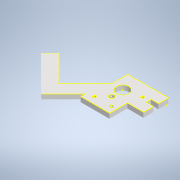
# Autodesk Inventor part: gripper laser cut
Saved by Autodesk Inventor 2020.1 (Build 241239000, 239)
## iProperties
Created: 2019-10-24
Part Number: gripper laser cut
Material: Generic
Document SubType Name: Modeling
Designer: amirs
Density: 1 g/cm^3
Appearance: Default
Author: amirs
Autodesk Inventor part; units mm, degrees
ref_plane "YZ Plane" through (0, 0, 0) normal (1, 0, 0) x (0, 1, 0)
ref_plane "XZ Plane" through (0, 0, 0) normal (0, 1, 0) x (-1, 0, 0)
ref_plane "XY Plane" through (0, 0, 0) normal (0, 0, 1) x (1, 0, 0)
sketch "Sketch1" plane through (0, 0, 0) normal (0, 1, 0) x (-1, 0, 0)
  line L0 (51.5704, 31.4309) -> (74.021, 53.8815)
  line L1 (74.021, 53.8815) -> (109.942, 17.9605)
  line L2 (109.942, 17.9605) -> (100.9618, 8.9803)
  line L3 (100.9618, 8.9803) -> (74.021, 35.921)
  line L4 (74.021, 35.921) -> (47.0803, 8.9803)
  line L5 (100.9618, 8.9803) -> (107.5624, 2.3796) construction
  line L6 (35.9043, 29.2241) -> (44.6165, 29.2241) construction
  line L7 (35.9043, 29.2241) -> (27.1921, 29.2241) construction
  circle A0 centre (44.6165, 29.2241) radius 1.5263
  circle A1 centre (27.1921, 29.2241) radius 1.6891
  circle A2 centre (35.9043, 20.4103) radius 2.54
  circle A3 centre (35.9043, 8.9803) radius 6.35
  line L8 (51.5704, 31.4309) -> (51.5704, 36.1902)
  line L9 (51.5704, 36.1902) -> (22.0986, 36.1902)
  line L10 (22.0986, 36.1902) -> (22.0986, 17.9605)
  line L11 (47.0803, 8.9803) -> (47.0803, 0)
  line L12 (5.5886, 17.9605) -> (22.0986, 17.9605)
  line L13 (5.5886, 17.9605) -> (5.5886, -7.4395)
  line L14 (5.5886, -7.4395) -> (47.0803, -7.4395)
  line L15 (47.0803, -7.4395) -> (47.0803, 0)
  point P0 (0, 0)
  dimension "d1" = 12.7
  dimension "d3" = 38.1
  dimension "d5" = 12.7
  dimension "d19" = 8.7122
  dimension "d20" = 8.7122
  dimension "d23" = 5.08
  dimension "d24" = 25.4
  dimension "d38" = 16.51
  dimension "d39" = 29.4718
  constraints: 32 end point, 7 perpendicular, 4 centre point, 3 vertical, 2 coincident, 2 horizontal, 1 parallel, 1 point on line
  measures "d1" distance between parallel lines of L4 L0
  measures "d3" distance of L2.end L3.end
  measures "d5" distance between parallel lines of L1 L3
  measures "d19" distance of L6.start L6.end
  measures "d20" distance of L6.start L7.end
  measures "d23" diameter of A2
  measures "d24" distance of L12.start L13.end
  measures "d38" distance of L12.start L10.end
  measures "d39" distance between parallel lines of L8 L10
extrude "Extrusion1" add sketch "Sketch1" along normal blind 5.08
sketch "Sketch2" plane through (0, 5.08, 0) normal (0, 1, 0) x (1, 0, 0)
  line L0 (-5.5886, -17.9605) -> (-5.5886, 7.4395) projected
  line L1 (-13.1234, -2.7205) -> (-13.1234, -7.8005)
  line L2 (-13.1234, -5.2605) -> (-2.9634, -5.2605) construction
  line L3 (-5.5886, 7.4395) -> (-47.0803, 7.4395) construction
  line L4 (-22.0986, -17.9605) -> (-5.5886, -17.9605) construction
  line L5 (-13.1234, -7.8005) -> (-2.9634, -7.8005)
  line L6 (-2.9634, -7.8005) -> (-2.9634, -2.7205)
  line L7 (-2.9634, -2.7205) -> (-13.1234, -2.7205)
  line L8 (-13.1234, -2.7205) -> (-13.1234, -7.8005)
  line L9 (-47.0803, 7.4395) -> (-47.0803, -8.9803) projected
  point P0 (0, 0)
  point P1 (-5.5886, -2.7205)
  point P2 (-5.5886, -7.8005)
  dimension "d29" = 5.08
  dimension "d30" = 12.7
  dimension "d31" = 25.4
  dimension "d40" = 33.9568
  dimension "d41" = 10.16
  constraints: 12 end point, 2 parallel, 1 horizontal, 1 midpoint, 1 perpendicular, 1 other
  measures "d29" distance of L1.start L1.end
  measures "d30" distance between parallel lines of L3 L2
  measures "d31" distance between parallel lines of L4 L3
  measures "d40" distance between parallel lines of L9 L1
  measures "d41" distance between parallel lines of L6 L1
extrude "Extrusion2" cut sketch "Sketch2" against normal blind 25.4 contours L5 L1 L7 L0
sketch "Sketch3" plane through (0, 5.08, 0) normal (0, 1, 0) x (1, 0, 0)
  circle A0 centre (-19.4734, -5.2605) radius 1.4605
  line L0 (-13.1234, -7.8005) -> (-13.1234, -2.7205) projected
  line L1 (-13.1234, -5.2605) -> (-2.0744, -5.2605) construction
  point P0 (0, 0)
  dimension "d34" = 6.35
  dimension "d35" = 2.921
  constraints: 2 end point, 2 midpoint, 1 centre point, 1 horizontal, 1 horizontal alignment
  measures "d34" distance from line of L0 A0.centre
  measures "d35" diameter of A0
extrude "Extrusion3" cut sketch "Sketch3" against normal blind 25.4
sketch "Sketch4" plane through (0, 5.08, 0) normal (0, 1, 0) x (1, 0, 0)
  circle A0 centre (-19.4734, -5.2605) radius 1.4605 projected
  line L0 (-13.1234, -2.7205) -> (-5.5886, -2.7205) projected
  line L1 (-5.5886, -2.7205) -> (-5.5886, 7.4395) projected
  line L2 (-5.5886, 7.4395) -> (-47.0803, 7.4395) projected
  line L3 (-47.0803, 7.4395) -> (-47.0803, -8.9803) projected
  line L4 (-47.0803, -8.9803) -> (-74.021, -35.921) projected
  line L5 (-74.021, -35.921) -> (-100.9618, -8.9803) projected
  line L6 (-100.9618, -8.9803) -> (-109.942, -17.9605) projected
  line L7 (-109.942, -17.9605) -> (-74.021, -53.8815) projected
  line L8 (-74.021, -53.8815) -> (-51.5704, -31.4309) projected
  line L9 (-51.5704, -31.4309) -> (-51.5704, -36.1902) projected
  line L10 (-51.5704, -36.1902) -> (-22.0986, -36.1902) projected
  line L11 (-22.0986, -36.1902) -> (-22.0986, -17.9605) projected
  line L12 (-22.0986, -17.9605) -> (-5.5886, -17.9605) projected
  line L13 (-5.5886, -17.9605) -> (-5.5886, -7.8005) projected
  line L14 (-5.5886, -7.8005) -> (-13.1234, -7.8005) projected
  line L15 (-13.1234, -7.8005) -> (-13.1234, -2.7205) projected
  circle A1 centre (-44.6165, -29.2241) radius 1.5263 projected
  circle A2 centre (-27.1921, -29.2241) radius 1.6891 projected
  circle A3 centre (-35.9043, -20.4103) radius 2.54 projected
  circle A4 centre (-35.9043, -8.9803) radius 6.35 projected
  point P0 (0, 0)
body "Solid1"
